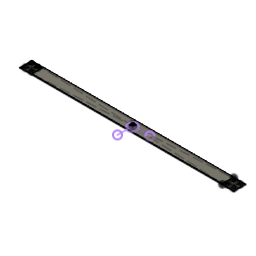
mobius strip v1 (Autodesk Fusion 360 design; units mm, degrees)
Autodesk Fusion 360 part; units mm, degrees
sketch "Sketch1" plane through (0, 0, 0) normal (0, 1, 0) x (1, 0, 0)
  line L0 (140, -7.5) -> (-140, -7.5)
  line L1 (-140, -7.5) -> (-140, 7.5)
  line L2 (-140, 7.5) -> (140, 7.5)
  line L3 (140, 7.5) -> (140, -7.5)
  line L4 (140, -7.5) -> (-140, 7.5) construction
  line L5 (-140, -7.5) -> (140, 7.5) construction
  line L6 (-125, 7.5) -> (-125, -7.5)
  line L7 (-140, 7.5) -> (-125, -7.5) construction
  line L8 (-125, 7.5) -> (-140, -7.5) construction
  circle A0 centre (-136.4645, 3.9645) radius 1.5
  circle A1 centre (-128.5355, 3.9645) radius 1.5
  line L9 (1.75, 0) -> (22.5, 0)
  circle A2 centre (-136.4645, -3.9645) radius 1.5
  circle A3 centre (-128.5355, -3.9645) radius 1.5
  line L10 (0, -20) -> (0, -2.5)
  line L11 (125, 7.5) -> (125, -7.5)
  circle A4 centre (128.5355, 3.9645) radius 1.5
  circle A5 centre (128.5355, -3.9645) radius 1.5
  circle A6 centre (136.4645, -3.9645) radius 1.5
  circle A7 centre (136.4645, 3.9645) radius 1.5
  dimension "d1" = 280
  dimension "d2" = 15
  dimension "d3" = 15
  dimension "d4" = 3
  dimension "d5" = 3
  dimension "d6" = 5
  dimension "d7" = 5
  constraint horizontal L0
  constraint perpendicular L0 L1
  constraint parallel L0 L2
  constraint parallel L1 L3
  constraint coincident L4 origin
  constraint coincident L5 origin
  constraint coincident L2 L6.start
  constraint coincident L0 L6.end
  constraint perpendicular L0 L6
  constraint coincident L7 A0.centre
  constraint coincident L8 A1.centre
  constraint symmetric A0 L9 A2
  constraint symmetric A1 L9 A3
  constraint symmetric L6.start L10 L11.start
  constraint symmetric L6.end L10 L11.end
  constraint symmetric A0 L10 A7
  constraint symmetric A1 L10 A4
  constraint symmetric A2 L10 A6
  constraint symmetric A3 L10 A5
  measures "d1" distance of L1.end L2.end
  measures "d2" distance of L0.end L1.end
  measures "d3" distance of L1 L6
  measures "d4" diameter of A0
  measures "d5" diameter of A1
  measures "d6" distance of L6.start A1.centre
  measures "d7" distance of L1.end A0.centre
extrude "Extrude1" add sketch "Sketch1" along normal blind 0.9 contours L0 L2 L6 L11
extrude "Extrude2" add sketch "Sketch1" along normal blind 0.45 contours L0 L2 L3 L11 | L0 L1 L2 L6
extrude "Extrude3" add sketch "Sketch1" along normal blind 2 contours A0 | A2 | A6 | A7
move_face "OffsetFaces1" offset -0.2 2 faces at (140, 0.15, -2.5) (-140, 0.15, 2.5)
named bodies: "mobius strip"
